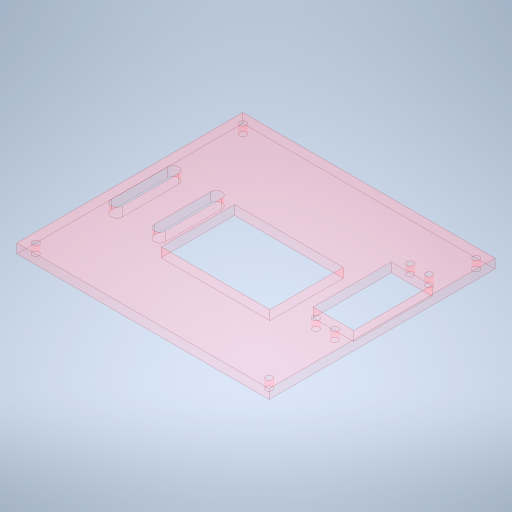
# Autodesk Inventor part: top_plate
Saved by Autodesk Inventor 2024 (Build 280153000, 153)
## iProperties
Created: 2024-01-24
Part Number: top_plate
Material: Generic
Document SubType Name: Modeling
Designer: critt
Density: 1 g/cm^3
Appearance: Default
Author: critt
## iProperties of the stored document tamiya_chassis_3DPrint.ipt
Created: 2024-01-26
Part Number: tamiya_chassis_3DPrint
Material: Generic
Document SubType Name: Modeling
Designer: critt
Density: 1 g/cm^3
Appearance: Default
Author: critt
Autodesk Inventor part; units mm, degrees
ref_plane "YZ Plane" through (0, 0, 0) normal (1, 0, 0) x (0, 1, 0)
ref_plane "XZ Plane" through (0, 0, 0) normal (0, 1, 0) x (-1, 0, 0)
ref_plane "XY Plane" through (0, 0, 0) normal (0, 0, 1) x (1, 0, 0)
sketch "Sketch20" plane through (0, 0, 0) normal (0, 1, 0) x (-1, 0, 0)
  line L0 (0, 0) -> (181, 0)
  line L1 (181, 0) -> (181, 120)
  line L2 (181, 120) -> (0, 120)
  line L3 (0, 120) -> (0, 0)
  point P0 (90.5, 120)
  dimension "d122" = 181
  dimension "d123" = 120
  constraints: 8 end point, 2 parallel, 1 horizontal, 1 midpoint, 1 perpendicular
  measures "d122" distance of L1.end L2.end
  measures "d123" distance from line of L0 point (90.5, 120)
extrude "Extrusion15" add sketch "Sketch20" along normal blind 5
sketch "Sketch22" plane through (0, 0, 0) normal (0, -1, 0) x (1, 0, 0)
  line L0 (-25.1, 70.1) -> (-5, 70.1)
  line L1 (-5, 70.1) -> (-5, 30)
  line L2 (-5, 30) -> (-25.1, 30)
  line L3 (-25.1, 30) -> (-25.1, 70.1)
  circle A0 centre (-15.05, 60) radius 1 construction
  line L4 (0, 120) -> (0, 0) construction
  circle A1 centre (-20.05, 25) radius 1.8
  circle A2 centre (-10.05, 25) radius 1.8
  circle A3 centre (-20.05, 75.1) radius 1.8
  circle A4 centre (-10.05, 75.1) radius 1.8
  line L5 (-15.05, 60) -> (0, 60) construction
  dimension "d126" = 40.1
  dimension "d127" = 20.1
  dimension "d128" = 2
  dimension "d129" = 30
  dimension "d130" = 10.05
  dimension "d134" = 5
  dimension "d135" = 5
  dimension "d136" = -5
  dimension "d137" = 5
  dimension "d138" = 5.05
  dimension "d139" = 5.05
  dimension "d140" = 5.05
  dimension "d141" = 5.05
  dimension "d142" = 3.6
  dimension "d159" = 15.05
  constraints: 10 end point, 5 centre point, 3 equal radius, 2 horizontal, 2 parallel, 1 midpoint, 1 perpendicular
  measures "d126" distance between parallel lines of L2 L0
  measures "d127" distance of L0.start L0.end
  measures "d128" diameter of A0
  measures "d129" distance from line of L2 L5.start
  measures "d130" distance from line of L1 L5.start
  measures "d134" distance from line of L2 A2.centre
  measures "d135" distance from line of L2 A1.centre
  measures "d136" distance from line of L0 A4.centre
  measures "d137" distance from line of L0 A3.centre
  measures "d138" distance from line of A1.centre L3
  measures "d139" distance from line of L1 A2.centre
  measures "d140" distance from line of L3 A3.centre
  measures "d141" distance from line of A4.centre L1
  measures "d142" diameter of A2
  measures "d159" distance of L5.start L5.end
extrude "Extrusion16" cut sketch "Sketch22" against normal blind 5
sketch "Sketch25" plane through (0, 0, 0) normal (0, -1, 0) x (1, 0, 0)
  line L0 (-181, 0) -> (-181, 120) projected
  line L1 (0, 0) -> (-181, 0) projected
  line L2 (-181, 120) -> (-134, 120)
  line L3 (-134, 120) -> (-134, 0)
  line L4 (-134, 0) -> (-181, 0)
  line L5 (-181, 0) -> (-181, 120)
  dimension "d150" = 47
  constraints: 8 end point, 2 parallel, 1 horizontal, 1 perpendicular, 1 point on line
  measures "d150" distance between parallel lines of L0 L3
extrude "Extrusion18" cut sketch "Sketch25" against normal blind 5
sketch "Sketch24" plane through (0, 0, 0) normal (0, -1, 0) x (1, 0, 0)
  circle A0 centre (-5, 5) radius 1.8
  circle A1 centre (-5, 115) radius 1.8
  circle A2 centre (-129, 115) radius 1.8
  circle A3 centre (-129, 5) radius 1.8
  line L0 (0, 0) -> (-181, 0) projected
  line L1 (0, 120) -> (0, 0) projected
  line L2 (-181, 120) -> (0, 120) projected
  circle A4 centre (-20.05, 25) radius 1.8 projected
  circle A5 centre (-10.05, 25) radius 1.8 projected
  circle A6 centre (-10.05, 75.1) radius 1.8 projected
  line L3 (-5, 70.1) -> (-5, 30) projected
  line L4 (-5, 30) -> (-25.1, 30) projected
  line L5 (-25.1, 30) -> (-25.1, 70.1) projected
  line L6 (-25.1, 70.1) -> (-5, 70.1) projected
  circle A7 centre (-20.05, 75.1) radius 1.8 projected
  line L7 (0, 0) -> (-134, 0) projected
  line L8 (0, 120) -> (0, 0) projected
  line L9 (-134, 120) -> (0, 120) projected
  line L10 (-134, 120) -> (-134, 0) projected
  dimension "d143" = 5
  dimension "d144" = 5
  dimension "d145" = 3.6
  dimension "d146" = 5
  dimension "d147" = 5
  dimension "d154" = 5
  dimension "d156" = 5
  dimension "d157" = 5
  dimension "d158" = 5
  constraints: 4 centre point, 3 equal radius
  measures "d143" distance from line of L0 A0.centre
  measures "d144" distance from line of A0.centre L1
  measures "d145" diameter of A0
  measures "d146" distance from line of L2 A1.centre
  measures "d147" distance from line of A1.centre L1
  measures "d154" distance from line of L2 A2.centre
  measures "d156" distance from line of L0 A3.centre
  measures "d157" distance from line of L10 A2.centre
  measures "d158" distance from line of L10 A3.centre
extrude "Extrusion17" cut sketch "Sketch24" against normal blind 5 contours A0 | A1 | A2 | A3
sketch "Sketch26" plane through (0, 0, 0) normal (0, -1, 0) x (1, 0, 0)
  circle A0 centre (-5, 5) radius 1.8 projected
  circle A1 centre (-129, 5) radius 1.8 projected
  circle A2 centre (-5, 115) radius 1.8 projected
  circle A3 centre (-129, 115) radius 1.8 projected
  line L0 (-134, 120) -> (-134, 0) projected
  line L1 (0, 0) -> (-134, 0) projected
  line L2 (0, 120) -> (0, 0) projected
  line L3 (-134, 120) -> (0, 120) projected
  circle A4 centre (-20.05, 25) radius 1.8 projected
  circle A5 centre (-10.05, 25) radius 1.8 projected
  circle A6 centre (-10.05, 75.1) radius 1.8 projected
  line L4 (-5, 70.1) -> (-5, 30) projected
  line L5 (-5, 30) -> (-25.1, 30) projected
  line L6 (-25.1, 30) -> (-25.1, 70.1) projected
  line L7 (-25.1, 70.1) -> (-5, 70.1) projected
  circle A7 centre (-20.05, 75.1) radius 1.8 projected
  line L8 (-4.5, 70.6) -> (-4.5, 29.5)
  line L9 (-4.5, 29.5) -> (-25.6, 29.5)
  line L10 (-25.6, 29.5) -> (-25.6, 70.6)
  line L11 (-25.6, 70.6) -> (-4.5, 70.6)
  dimension "d176" = 0.5
  constraints: 8 end point, 3 other
  measures "d176" distance between parallel lines of L9 L5
extrude "Extrusion19" cut sketch "Sketch26" against normal blind 25.4 contours L4 L5 L6 L7 | L8 L9 L10 L11
sketch "Sketch28" plane through (0, 5, 0) normal (0, 1, 0) x (1, 0, 0)
  line L0 (-49, -83.3) -> (-81, -83.3) projected
  arc A0 (-85, -79.3) -> (-81, -83.3) centre (-81, -79.3) ccw projected
  line L1 (-85, -79.3) -> (-85, -47.3) projected
  arc A1 (-81, -43.3) -> (-85, -47.3) centre (-81, -47.3) ccw projected
  line L2 (-81, -43.3) -> (-49, -43.3) projected
  arc A2 (-45, -47.3) -> (-49, -43.3) centre (-49, -47.3) ccw projected
  line L3 (-45, -47.3) -> (-45, -79.3) projected
  arc A3 (-49, -83.3) -> (-45, -79.3) centre (-49, -79.3) ccw projected
  line L4 (-81, -88.38) -> (-49, -88.38)
  arc A4 (-49, -88.38) -> (-39.92, -79.3) centre (-49, -79.3) ccw
  line L5 (-39.92, -79.3) -> (-39.92, -47.3)
  arc A5 (-39.92, -47.3) -> (-49, -38.22) centre (-49, -47.3) ccw
  line L6 (-49, -38.22) -> (-81, -38.22)
  arc A6 (-81, -38.22) -> (-90.08, -47.3) centre (-81, -47.3) ccw
  line L7 (-90.08, -47.3) -> (-90.08, -79.3)
  arc A7 (-90.08, -79.3) -> (-81, -88.38) centre (-81, -79.3) ccw
  point P0 (0, 0)
  dimension "d165" = 5.08
  constraints: 8 end point, 8 point on circle, 4 centre point, 7 other
  measures "d165" distance between parallel lines of L0 L4
extrude "Extrusion21" cut sketch "Sketch28" against normal blind 25.4 contours L0 A0 L1 A1 L2 A2 L3 A3 | A7 L7 A6 L6 A5 L5 A4 L4
sketch "Sketch29" plane through (0, 5, 0) normal (0, 1, 0) x (1, 0, 0)
  arc A0 (-106.08, -75) -> (-100.08, -75) centre (-103.08, -75) ccw
  line L0 (-100.08, -45) -> (-100.08, -75)
  line L1 (-106.08, -75) -> (-106.08, -45)
  arc A1 (-129, -75) -> (-123, -75) centre (-126, -75) ccw
  line L2 (-123, -45) -> (-123, -75)
  line L3 (-129, -75) -> (-129, -45)
  arc A2 (-123, -45) -> (-129, -45) centre (-126, -45) ccw
  arc A3 (-100.08, -45) -> (-106.08, -45) centre (-103.08, -45) ccw
  line L4 (-39.92, -47.3) -> (-39.92, -79.3) projected
  arc A4 (-49, -88.38) -> (-39.92, -79.3) centre (-49, -79.3) ccw projected
  line L5 (-49, -88.38) -> (-81, -88.38) projected
  arc A5 (-90.08, -79.3) -> (-81, -88.38) centre (-81, -79.3) ccw projected
  line L6 (-90.08, -79.3) -> (-90.08, -47.3) projected
  arc A6 (-81, -38.22) -> (-90.08, -47.3) centre (-81, -47.3) ccw projected
  line L7 (-81, -38.22) -> (-49, -38.22) projected
  arc A7 (-39.92, -47.3) -> (-49, -38.22) centre (-49, -47.3) ccw projected
  line L8 (-25.6, -29.5) -> (-4.5, -29.5) projected
  line L9 (-4.5, -29.5) -> (-4.5, -70.6) projected
  line L10 (-4.5, -70.6) -> (-25.6, -70.6) projected
  line L11 (-25.6, -70.6) -> (-25.6, -29.5) projected
  circle A8 centre (-5, -5) radius 1.8 projected
  circle A9 centre (-129, -5) radius 1.8 projected
  circle A10 centre (-5, -115) radius 1.8 projected
  circle A11 centre (-129, -115) radius 1.8 projected
  line L12 (-134, 0) -> (-134, -120) projected
  line L13 (-134, -120) -> (0, -120) projected
  line L14 (0, -120) -> (0, 0) projected
  line L15 (0, 0) -> (-134, 0) projected
  circle A12 centre (-20.05, -75.1) radius 1.8 projected
  circle A13 centre (-10.05, -75.1) radius 1.8 projected
  circle A14 centre (-10.05, -25) radius 1.8 projected
  circle A15 centre (-20.05, -25) radius 1.8 projected
  line L16 (-129, -60) -> (-134, -60) construction
  line L17 (-106.08, -60) -> (-123, -60) construction
  line L18 (-129, -45) -> (-126, -45) construction
  line L19 (-103.08, -45) -> (-106.08, -45) construction
  dimension "d139" = 5.05
  dimension "d168" = 30
  dimension "d169" = 5
  dimension "d170" = 10
  dimension "d171" = 6
  dimension "d172" = 6
  dimension "d173" = 3
  constraints: 16 end point, 8 point on circle, 4 centre point, 4 horizontal, 4 midpoint, 4 vertical, 3 equal radius, 3 parallel
  measures "d168" distance of L3.start L3.end
  measures "d169" distance of L16.start L16.end
  measures "d170" distance between parallel lines of L6 L0
  measures "d171" distance between parallel lines of L3 L2
  measures "d172" distance between parallel lines of L1 L0
  measures "d173" radius of A2
extrude "Extrusion22" cut sketch "Sketch29" against normal blind 25.4 contours L1 A3 L0 A0 | L3 A2 L2 A1
sketch "Sketch30" plane through (0, 5, 0) normal (0, 1, 0) x (1, 0, 0)
  arc A0 (-100.08, -45) -> (-106.08, -45) centre (-103.08, -45) ccw projected
  line L0 (-100.08, -45) -> (-100.08, -75) projected
  arc A1 (-106.08, -75) -> (-100.08, -75) centre (-103.08, -75) ccw projected
  line L1 (-106.08, -75) -> (-106.08, -45) projected
  arc A2 (-123, -45) -> (-129, -45) centre (-126, -45) ccw projected
  line L2 (-123, -45) -> (-123, -75) projected
  arc A3 (-129, -75) -> (-123, -75) centre (-126, -75) ccw projected
  line L3 (-129, -75) -> (-129, -45) projected
  line L4 (-39.92, -47.3) -> (-39.92, -79.3) projected
  arc A4 (-49, -88.38) -> (-39.92, -79.3) centre (-49, -79.3) ccw projected
  line L5 (-49, -88.38) -> (-81, -88.38) projected
  arc A5 (-90.08, -79.3) -> (-81, -88.38) centre (-81, -79.3) ccw projected
  line L6 (-90.08, -79.3) -> (-90.08, -47.3) projected
  arc A6 (-81, -38.22) -> (-90.08, -47.3) centre (-81, -47.3) ccw projected
  line L7 (-81, -38.22) -> (-49, -38.22) projected
  arc A7 (-39.92, -47.3) -> (-49, -38.22) centre (-49, -47.3) ccw projected
  line L8 (-25.6, -29.5) -> (-4.5, -29.5) projected
  line L9 (-4.5, -29.5) -> (-4.5, -70.6) projected
  line L10 (-4.5, -70.6) -> (-25.6, -70.6) projected
  line L11 (-25.6, -70.6) -> (-25.6, -29.5) projected
  circle A8 centre (-5, -5) radius 1.8 projected
  circle A9 centre (-129, -5) radius 1.8 projected
  circle A10 centre (-5, -115) radius 1.8 projected
  circle A11 centre (-129, -115) radius 1.8 projected
  line L12 (-134, 0) -> (-134, -120) projected
  line L13 (-134, -120) -> (0, -120) projected
  line L14 (0, -120) -> (0, 0) projected
  line L15 (0, 0) -> (-134, 0) projected
  circle A12 centre (-20.05, -75.1) radius 1.8 projected
  circle A13 centre (-10.05, -75.1) radius 1.8 projected
  circle A14 centre (-10.05, -25) radius 1.8 projected
  circle A15 centre (-20.05, -25) radius 1.8 projected
extrude "Extrusion23" add sketch "Sketch30" against normal blind 5 contours L4 A4 L5 A5 L6 A6 L7 A7
sketch "Sketch31" plane through (0, 5, 0) normal (0, 1, 0) x (1, 0, 0)
  arc A0 (-100.08, -45) -> (-106.08, -45) centre (-103.08, -45) ccw projected
  line L0 (-100.08, -45) -> (-100.08, -75) projected
  arc A1 (-106.08, -75) -> (-100.08, -75) centre (-103.08, -75) ccw projected
  line L1 (-106.08, -75) -> (-106.08, -45) projected
  arc A2 (-123, -45) -> (-129, -45) centre (-126, -45) ccw projected
  line L2 (-123, -45) -> (-123, -75) projected
  arc A3 (-129, -75) -> (-123, -75) centre (-126, -75) ccw projected
  line L3 (-129, -75) -> (-129, -45) projected
  line L4 (-25.6, -29.5) -> (-4.5, -29.5) projected
  line L5 (-4.5, -29.5) -> (-4.5, -70.6) projected
  line L6 (-4.5, -70.6) -> (-25.6, -70.6) projected
  line L7 (-25.6, -70.6) -> (-25.6, -29.5) projected
  circle A4 centre (-5, -5) radius 1.8 projected
  circle A5 centre (-129, -5) radius 1.8 projected
  circle A6 centre (-5, -115) radius 1.8 projected
  circle A7 centre (-129, -115) radius 1.8 projected
  line L8 (-134, 0) -> (-134, -120) projected
  line L9 (-134, -120) -> (0, -120) projected
  line L10 (0, -120) -> (0, 0) projected
  line L11 (0, 0) -> (-134, 0) projected
  circle A8 centre (-20.05, -75.1) radius 1.8 projected
  circle A9 centre (-10.05, -75.1) radius 1.8 projected
  circle A10 centre (-10.05, -25) radius 1.8 projected
  circle A11 centre (-20.05, -25) radius 1.8 projected
  line L12 (-4.246, -29.246) -> (-25.854, -29.246)
  line L13 (-25.854, -29.246) -> (-25.854, -70.854)
  line L14 (-25.854, -70.854) -> (-4.246, -70.854)
  line L15 (-4.246, -70.854) -> (-4.246, -29.246)
  dimension "d179" = 0.254
  constraints: 8 end point, 3 other
  measures "d179" distance between parallel lines of L4 L12
extrude "Extrusion24" cut sketch "Sketch31" against normal blind 5 contours L4 L5 L6 L7 | L15 L14 L13 L12
sketch "Sketch32" plane through (0, 5, 0) normal (0, 1, 0) x (1, 0, 0)
  line L0 (-93.9, -44.81) -> (-93.9, -83.21) projected
  line L1 (-93.9, -83.51) -> (-36.1, -83.51) projected
  line L2 (-93.9, -83.51) -> (-36.1, -83.51) projected
  line L3 (-36.1, -83.21) -> (-36.1, -44.81) projected
  line L4 (-93.9, -83.21) -> (-36.1, -83.21) projected
  line L5 (-36.1, -44.81) -> (-93.9, -44.81) projected
  line L6 (-36.1, -44.51) -> (-93.9, -44.51) projected
  line L7 (-36.1, -44.51) -> (-93.9, -44.51) projected
  line L8 (-36.1, -83.51) -> (-93.9, -83.51)
  line L9 (-93.9, -83.51) -> (-93.9, -44.51)
  line L10 (-93.9, -44.51) -> (-36.1, -44.51)
  line L11 (-36.1, -44.51) -> (-36.1, -83.51)
  point P0 (0, 0)
  constraints: 8 end point, 2 parallel, 1 horizontal, 1 perpendicular
extrude "Extrusion25" cut sketch "Sketch32" against normal blind 5
body "Solid2"
